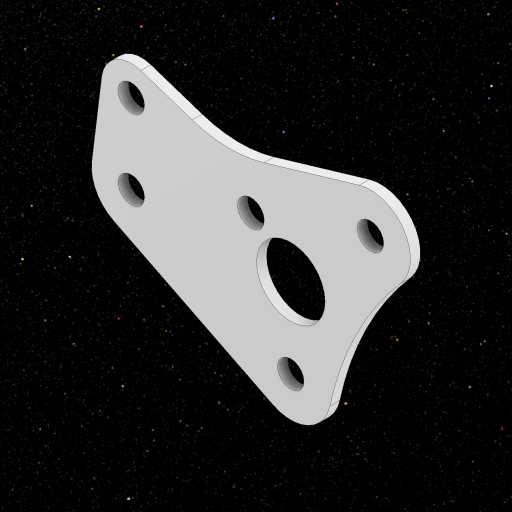
# Autodesk Inventor part: gearbox_gusset
Saved by Autodesk Inventor 2024 (Build 280153000, 153)
## iProperties
Created: 2024-02-16
Part Number: gearbox_gusset
Material: Acetal Resin, White
Document SubType Name: Modeling
Designer: Averey Ku
Density: 1.425 g/cm^3
Appearance: Smooth - White
Author: Averey Ku
Autodesk Inventor part; units mm, degrees
ref_plane "YZ Plane" through (0, 0, 0) normal (1, 0, 0) x (0, 1, 0)
ref_plane "XZ Plane" through (0, 0, 0) normal (0, 1, 0) x (-1, 0, 0)
ref_plane "XY Plane" through (0, 0, 0) normal (0, 0, 1) x (1, 0, 0)
sketch "Sketch1" plane through (0, 0, 0) normal (0, 0, 1) x (1, 0, 0)
  circle A0 centre (0, 0) radius 2.0955
  circle A1 centre (0, 12.7) radius 2.0955
  circle A2 centre (19.05, 6.35) radius 2.1209
  circle A3 centre (38.1, 12.7) radius 2.0955
  circle A4 centre (25.4, -12.7) radius 2.0955
  arc A5 (-6.3002, 0.7937) -> (-2.8398, -5.6796) centre (0, 0) ccw
  arc A6 (1.506, 17.2181) -> (-4.7251, 13.2953) centre (0, 12.7) ccw
  arc A7 (42.896, 8.5381) -> (36.3, 18.7895) centre (38.1, 12.7) ccw
  arc A8 (22.5602, -18.3796) -> (31.7002, -13.4938) centre (25.4, -12.7) ccw
  circle A9 centre (25.4, 0) radius 5.461
  line L0 (9.6793, 14.4937) -> (1.506, 17.2181)
  line L1 (36.3, 18.7895) -> (21.1035, 14.2975)
  arc A10 (9.6793, 14.4937) -> (21.1035, 14.2975) centre (15.7034, 32.5661) ccw
  arc A11 (42.896, 8.5381) -> (31.6071, -14.0397) centre (81.2637, -24.7569) ccw
  line L2 (-4.7251, 13.2953) -> (-6.3002, 0.7937)
  line L3 (-2.8398, -5.6796) -> (22.5602, -18.3796)
  point P0 (40.6465, 18.517)
  point P1 (44.45, 12.7)
  dimension "d0" = 4.191
  dimension "d1" = 4.191
  dimension "d2" = 4.2418
  dimension "d3" = 4.191
  dimension "d4" = 4.191
  dimension "d5" = 12.7
  dimension "d9" = 10.922
  dimension "d10" = 19.05
  dimension "d16" = 6.35
  constraints: 15 point on circle, 12 centre point, 10 tangent, 8 end point, 5 coincident, 3 other
  measures "d0" diameter of A0
  measures "d1" diameter of A1
  measures "d2" diameter of A2
  measures "d3" diameter of A3
  measures "d4" diameter of A4
  measures "d5" diameter of A5
  measures "d9" diameter of A9
  measures "d10" radius of A10
  measures "d16" radius of A7
extrude "Extrusion1" add sketch "Sketch1" along normal blind 1.5875
body "Solid1"
